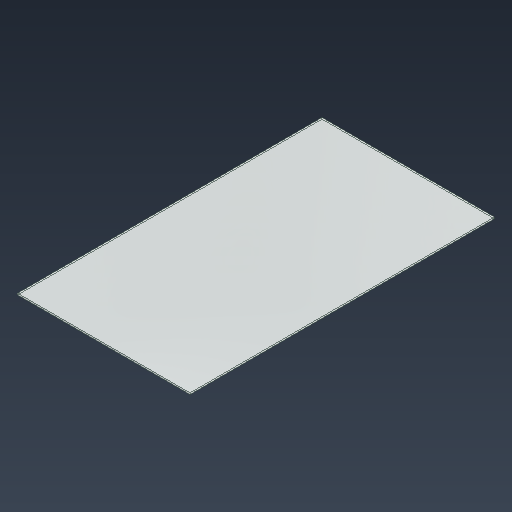
# Autodesk Inventor part: glassPlate
Saved by Autodesk Inventor 2021 (Build 250183000, 183)
## iProperties
Created: 2021-11-24
Part Number: glassPlate
Material: Generic
Document SubType Name: Modeling
Designer: jo_ki
Density: 1 g/cm^3
Appearance: Clear
Author: jo_ki
Autodesk Inventor part; units mm, degrees
ref_plane "YZ Plane" through (0, 0, 0) normal (1, 0, 0) x (0, 1, 0)
ref_plane "XZ Plane" through (0, 0, 0) normal (0, 1, 0) x (-1, 0, 0)
ref_plane "XY Plane" through (0, 0, 0) normal (0, 0, 1) x (1, 0, 0)
derived "Mastersketch.ipt"
sketch "Sketch2" plane through (0, 0, 0) normal (0, 1, 0) x (-1, 0, 0)
  line L0 (-340, 600) -> (340, 600)
  line L1 (340, 600) -> (340, -600)
  line L2 (340, -600) -> (-340, -600)
  line L3 (-340, -600) -> (-340, 600)
  line L4 (-340, 600) -> (340, -600) construction
  line L5 (340, 600) -> (-340, -600) construction
  point P0 (0, 0)
  dimension "d1" = 1200
  dimension "d2" = 680
  constraints: 12 end point, 2 midpoint, 2 parallel, 1 horizontal, 1 perpendicular
  measures "d1" distance between parallel lines of L0 L2
  measures "d2" distance of L1.end L2.end
extrude "Extrusion1" add sketch "Sketch2" along normal blind 6
equation "\"d1\" = glass_length"
equation "\"d2\" = feet_widthCenter - profile_width"
equation "\"d3\" = glass_thickness"
equation "\"glass_length\" = 1200"
equation "\"feet_widthCenter\" = 720"
equation "\"profile_width\" = 40"
equation "\"glass_thickness\" = 6"
body "Solid1"
